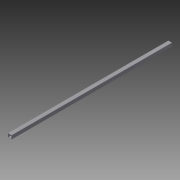
# Autodesk Inventor part: Frame0002
Saved by Autodesk Inventor 2013 (Build 170138000, 138)
## iProperties
Created: 2013-01-13
Part Number: Frame0002
Material: Generic
Document SubType Name: Modeling
Designer: Phillip
Density: 1 g/cm^3
d0: 1.750 in
d1: 1.750 in
d2: 0.125 in
d3: 78.000 in
d4: 0.00 deg
Author: Phillip
Autodesk Inventor part; units mm, degrees
ref_plane "YZ Plane" through (0, 0, 0) normal (1, 0, 0) x (0, 1, 0)
ref_plane "XZ Plane" through (0, 0, 0) normal (0, 1, 0) x (-1, 0, 0)
ref_plane "XY Plane" through (0, 0, 0) normal (0, 0, 1) x (1, 0, 0)
sketch "Sketch1" plane through (0, 0, 0) normal (0, 0, 1) x (1, 0, 0)
  line L0 (22.225, -22.225) -> (-22.225, -22.225)
  line L1 (-22.225, -22.225) -> (-22.225, 22.225)
  line L2 (-22.225, 22.225) -> (22.225, 22.225)
  line L3 (22.225, 22.225) -> (22.225, -22.225)
  line L4 (-19.05, -19.05) -> (19.05, -19.05)
  line L5 (19.05, -19.05) -> (19.05, 19.05)
  line L6 (19.05, 19.05) -> (-19.05, 19.05)
  line L7 (-19.05, 19.05) -> (-19.05, -19.05)
  point P0 (0, 0)
  point P1 (0, 22.225)
  point P2 (22.225, 0)
  dimension "d0" = 44.45
  dimension "d1" = 44.45
  dimension "d2" = 3.175
  constraints: 16 end point, 4 parallel, 2 midpoint, 2 perpendicular, 1 horizontal, 1 horizontal alignment, 1 vertical alignment, 3 other
  measures "d0" distance of L1.end L2.end
  measures "d1" distance of L2.end L0.start
  measures "d2" distance between parallel lines of L0 L4
extrude "Extrusion1" add sketch "Sketch1" along normal blind 1981.2
body "Solid1"
